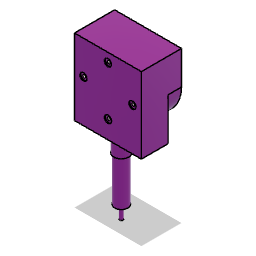
Braço robótico 3.0 (suporte para o braço) v14 (Autodesk Fusion 360 design; units mm, degrees)
Autodesk Fusion 360 part; units mm, degrees
sketch "Sketch1" plane through (0, 0, 0) normal (0, 0, 1) x (1, 0, 0)
  line L0 (-37.5, 0) -> (-37.5, 37.5)
  line L1 (-37.5, 37.5) -> (37.5, 37.5)
  line L2 (37.5, 37.5) -> (37.5, 0)
  arc A0 (-37.5, 0) -> (37.5, 0) centre (0, 0) ccw
  dimension "d1" = 75
  dimension "d2" = 75
  constraint parallel L0 L2
  measures "d1" diameter of A0
  measures "d2" distance of L0.end L1.end
extrude "Extrude1" add sketch "Sketch1" along normal blind 35
sketch "Sketch2" plane through (0, 37.5, 0) normal (0, 1, 0) x (-1, 0, 0)
  line L0 (-37.5, 0) -> (37.5, 0)
  line L1 (37.5, 0) -> (37.5, 35)
  line L2 (37.5, 35) -> (-37.5, 35)
  line L3 (-37.5, 35) -> (-37.5, 0)
  line L4 (37.5, 65) -> (-37.5, 65)
  line L5 (-37.5, 65) -> (-37.5, 25)
  line L6 (-37.5, 25) -> (37.5, 25)
  line L7 (37.5, 25) -> (37.5, 65)
  line L8 (37.5, 65) -> (-37.5, 25) construction
  line L9 (-37.5, 65) -> (37.5, 25) construction
  point P0 (0, 45)
  dimension "d6" = 75
  dimension "d7" = 40
  constraint horizontal L4
  constraint perpendicular L4 L5
  constraint parallel L4 L6
  constraint parallel L5 L7
  constraint coincident L8 P0
  constraint coincident L9 P0
  measures "d6" distance of L5.end L6.end
  measures "d7" distance of L4.end L5.end
extrude "Extrude2" add sketch "Sketch2" against normal blind 85 contours L2 L4 L5 L7
sketch "Sketch3" plane through (0, 0, 0) normal (0, 1, 0) x (1, 0, 0)
  circle A0 centre (0, -50) radius 8.5
  point P0 (0, -50)
  dimension "d12" = 17
  constraint coincident P0 A0.centre
  measures "d12" diameter of A0
extrude "Extrude3" add sketch "Sketch3" against normal blind 107.5
sketch "Sketch4" plane through (0, -107.5, 0) normal (0, -1, 0) x (1, 0, 0)
  circle A0 centre (0, 50) radius 8.5
  circle A1 centre (0, 50) radius 7.5
  dimension "d15" = 15
  constraint concentric A0 A1
  measures "d15" diameter of A1
extrude "Extrude4" cut sketch "Sketch4" against normal blind 40
sketch "Sketch5" plane through (0, 0, 0) normal (0, 0, -1) x (-1, 0, 0)
  line L0 (37.5, 0) -> (37.5, 37.5)
  line L1 (37.5, 37.5) -> (-37.5, 37.5)
  line L2 (-37.5, 37.5) -> (-37.5, 0)
  arc A0 (-37.5, 0) -> (37.5, 0) centre (0, 0) ccw
  line L3 (0, 37.5) -> (0, 27.5)
  line L4 (-37.5, 0) -> (-27.5, 0)
  line L5 (37.5, 0) -> (27.5, 0)
  line L6 (0, -37.5) -> (0, -27.5)
  dimension "d18" = 10
  dimension "d19" = 10
  dimension "d20" = 10
  dimension "d21" = 10
  constraint midpoint L1 L3.start
  constraint perpendicular L1 L3
  constraint coincident L2.end A0.start
  constraint perpendicular L2 L4
  constraint coincident L0.start A0.end
  constraint perpendicular L0 L5
  constraint midpoint A0 L6.start
  constraint parallel L2 L6
  measures "d18" distance of L3.start L3.end
  measures "d19" distance of L2.end L4.end
  measures "d20" distance of L0.start L5.end
  measures "d21" distance of L6.start L6.end
extrude "Extrude6" cut 1 faces at (-12.5, 25, 0) along direction (0, 0, 1) blind 20
sketch "Sketch6" plane through (0, -107.5, 0) normal (0, -1, 0) x (1, 0, 0)
  circle A0 centre (0, 50) radius 7.5
  circle A1 centre (0, 50) radius 7.5
  constraint concentric A0 A1
extrude "Extrude7" add sketch "Sketch6" along normal blind 10
sketch "Sketch7" plane through (0, -117.5, 0) normal (0, -1, 0) x (1, 0, 0)
  circle A0 centre (0, 50) radius 7.5
  circle A1 centre (0, 50) radius 2
  dimension "d33" = 4
  constraint concentric A0 A1
  measures "d33" diameter of A1
extrude "Extrude8" add sketch "Sketch7" along normal blind 14.509 contours A1
sketch "Sketch8" plane through (0, 0, 65) normal (0, 0, 1) x (1, 0, 0)
  line L0 (37.5, 37.5) -> (-37.5, 37.5)
  line L1 (-37.5, 37.5) -> (-37.5, -47.5)
  line L2 (-37.5, -47.5) -> (37.5, -47.5)
  line L3 (37.5, -47.5) -> (37.5, 37.5)
  line L4 (0, 37.5) -> (0, 27.5)
  line L5 (-37.5, 0) -> (-27.5, 0)
  line L6 (0, -37.5) -> (0, -27.5)
  line L7 (37.5, 0) -> (27.5, 0)
  dimension "d36" = 10
  dimension "d38" = 360
  constraint midpoint L0 L4.start
  constraint perpendicular L0 L4
  measures "d36" distance of L4.start L4.end
hole "Hole2" at (0, 27.5, 65) at (27.5, 0, 65) at (-27.5, 0, 65) at (0, -27.5, 65) direction (0, 0, -1) diameter 3.332 end through all counterbore diameter 8 counterbore depth 1
thread "Thread2" "ISO Metric profile 4.0 M4x0.7 6H"
